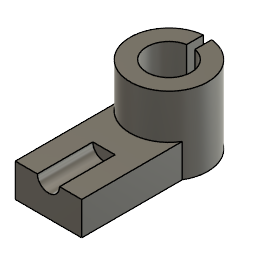
tr2 (Autodesk Fusion 360 design; units mm, degrees)
part number: 2026-08-20-00-14-58-411
Autodesk Fusion 360 part; units mm, degrees
sketch "Sketch1" plane through (0, 0, 0) normal (0, 1, 0) x (1, 0, 0)
  line L0 (-240, 275.7779) -> (-240, -450)
  line L1 (-240, -450) -> (240, -450)
  line L2 (240, -450) -> (240, 275.7779)
  line L3 (240, 450) -> (-240, -450) construction
  line L4 (-240, 450) -> (240, -450) construction
  line L5 (30, 577.1623) -> (30, 698.3882)
  line L6 (-30, 698.3882) -> (-30, 577.1623)
  arc A0 (-30, 698.3882) -> (30, 698.3882) centre (0, 420) ccw
  arc A1 (-30, 577.1623) -> (30, 577.1623) centre (0, 420) ccw
  dimension "d1" = 480
  dimension "d2" = 900
  dimension "d3" = 560
  dimension "d4" = 420
  dimension "d5" = 320
  constraint parallel L0 L2
  constraint coincident L3 origin
  constraint coincident L4 origin
  constraint concentric A0 A1
  constraint coincident L0.start A0
  constraint coincident L2.end A0
  measures "d1" distance of L0.end L1.end
  measures "d2" distance of L4.start L0.end
  measures "d3" diameter of A0
  measures "d4" distance of origin A0.centre
  measures "d5" diameter of A1
extrude "Extrude1" add sketch "Sketch1" along normal blind 560 contours L5 L6 A0 A1 makes body 1
extrude "Extrude2" add sketch "Sketch1" along normal blind 240 separate body contours L0 L1 L2 A0 makes body 2
sketch "Sketch2" plane through (0, 0, 450) normal (0, 0, 1) x (1, 0, 0)
  line L0 (-240, 0) -> (240, 0)
  line L1 (240, 0) -> (240, 240)
  line L2 (240, 240) -> (-240, 240)
  line L3 (-240, 240) -> (-240, 0)
  circle A0 centre (0, 240) radius 80
  dimension "d12" = 160
  constraint midpoint L2 A0.centre
  measures "d12" diameter of A0
extrude "Extrude3" cut sketch "Sketch2" against normal blind 400 contours L2 A0 picked at (-9.7424, 215.1767) bodies 2
combine "Combine1" operation add target body 1 tool bodies 2
